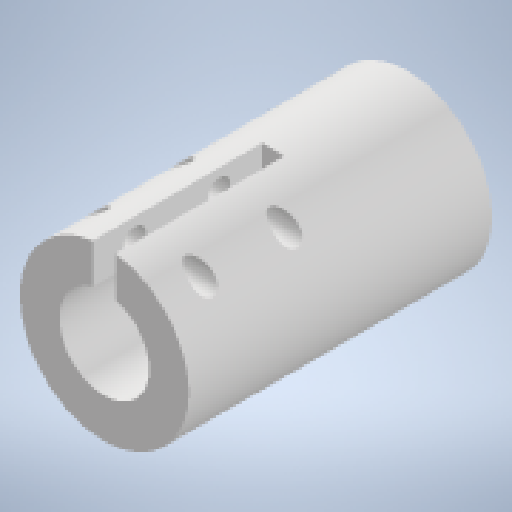
# Autodesk Inventor part: združevalnik_osi
Saved by Autodesk Inventor 2023 (Build 270158000, 158)
## iProperties
Created: 2022-09-16
Part Number: združevalnik_osi
Material: Generic
Document SubType Name: Modeling
Designer: simon
Density: 1 g/cm^3
Appearance: Default
Author: simon
Autodesk Inventor part; units mm, degrees
ref_plane "YZ Plane" through (0, 0, 0) normal (1, 0, 0) x (0, 1, 0)
ref_plane "XZ Plane" through (0, 0, 0) normal (0, 1, 0) x (-1, 0, 0)
ref_plane "XY Plane" through (0, 0, 0) normal (0, 0, 1) x (1, 0, 0)
sketch "Sketch1" plane through (0, 0, 0) normal (0, 0, 1) x (1, 0, 0)
  line L0 (-2.9047, -2.75) -> (-2.9047, 2.75) projected
  line L1 (-2.9047, 2.75) -> (2.9047, 2.75) projected
  line L2 (2.9047, 2.75) -> (2.9047, -2.75) projected
  line L3 (2.9047, -2.75) -> (-2.9047, -2.75) projected
  arc A0 (-7.5629, 23.8286) -> (-7.5205, 19.0707) centre (10.0684, 21.6064) ccw projected
  arc A1 (-7.5205, 19.0707) -> (-8.8044, 18.513) centre (0, 0) ccw projected
  arc A2 (-8.8044, 18.513) -> (-12.2528, 21.7915) centre (-22.663, 7.3892) ccw projected
  arc A3 (-12.2528, 21.7915) -> (-13.7113, 20.9046) centre (0, 0) ccw projected
  arc A4 (-13.7113, 20.9046) -> (-12.3868, 16.3345) centre (3.8657, 23.5216) ccw projected
  arc A5 (-12.3868, 16.3345) -> (-13.4727, 15.4511) centre (0, 0) ccw projected
  arc A6 (-13.4727, 15.4511) -> (-17.6777, 17.6777) centre (-23.8161, 1.0008) ccw projected
  arc A7 (-17.6777, 17.6777) -> (-18.8428, 16.4301) centre (0, 0) ccw projected
  arc A8 (-18.8428, 16.4301) -> (-16.3345, 12.3868) centre (-2.6237, 23.6923) ccw projected
  arc A9 (-16.3345, 12.3868) -> (-17.1417, 11.2433) centre (0, 0) ccw projected
  arc A10 (-17.1417, 11.2433) -> (-21.7915, 12.2528) centre (-23.203, -5.4619) ccw projected
  arc A11 (-21.7915, 12.2528) -> (-22.5769, 10.7371) centre (0, 0) ccw projected
  arc A12 (-22.5769, 10.7371) -> (-19.0707, 7.5205) centre (-8.9185, 22.1059) ccw projected
  arc A13 (-19.0707, 7.5205) -> (-19.5395, 6.2015) centre (0, 0) ccw projected
  arc A14 (-19.5395, 6.2015) -> (-24.2892, 5.9191) centre (-20.869, -11.5194) ccw projected
  arc A15 (-24.2892, 5.9191) -> (-24.6365, 4.2478) centre (0, 0) ccw projected
  arc A16 (-24.6365, 4.2478) -> (-20.3925, 2.0964) centre (-14.5519, 18.88) ccw projected
  arc A17 (-20.3925, 2.0964) -> (-20.488, 0.6999) centre (0, 0) ccw projected
  arc A18 (-20.488, 0.6999) -> (-24.9854, -0.8535) centre (-16.9872, -16.7226) ccw projected
  arc A19 (-24.9854, -0.8535) -> (-24.8689, -2.5566) centre (0, 0) ccw projected
  arc A20 (-24.8689, -2.5566) -> (-20.2019, -3.4832) centre (-19.106, 14.2538) ccw projected
  arc A21 (-20.2019, -3.4832) -> (-19.9171, -4.8537) centre (0, 0) ccw projected
  arc A22 (-19.9171, -4.8537) -> (-23.8286, -7.5629) centre (-11.8455, -20.6856) ccw projected
  arc A23 (-23.8286, -7.5629) -> (-23.257, -9.1714) centre (0, 0) ccw projected
  arc A24 (-23.257, -9.1714) -> (-18.513, -8.8044) centre (-22.2431, 8.5705) ccw projected
  arc A25 (-18.513, -8.8044) -> (-17.869, -10.0473) centre (0, 0) ccw projected
  arc A26 (-17.869, -10.0473) -> (-20.9046, -13.7113) centre (-5.8254, -23.1144) ccw projected
  arc A27 (-20.9046, -13.7113) -> (-19.9201, -15.1059) centre (0, 0) ccw projected
  arc A28 (-19.9201, -15.1059) -> (-15.4511, -13.4727) centre (-23.7306, 2.2515) ccw projected
  arc A29 (-15.4511, -13.4727) -> (-14.4957, -14.4957) centre (0, 0) ccw projected
  arc A30 (-14.4957, -14.4957) -> (-16.4301, -18.8428) centre (0.6268, -23.8289) ccw projected
  arc A31 (-16.4301, -18.8428) -> (-15.1059, -19.9201) centre (0, 0) ccw projected
  arc A32 (-15.1059, -19.9201) -> (-11.2433, -17.1417) centre (-23.4581, -4.2344) ccw projected
  arc A33 (-11.2433, -17.1417) -> (-10.0473, -17.869) centre (0, 0) ccw projected
  arc A34 (-10.0473, -17.869) -> (-10.7371, -22.5769) centre (7.0326, -22.7762) ccw projected
  arc A35 (-10.7371, -22.5769) -> (-9.1714, -23.257) centre (0, 0) ccw projected
  arc A36 (-9.1714, -23.257) -> (-6.2015, -19.5395) centre (-21.4457, -10.4063) ccw projected
  arc A37 (-6.2015, -19.5395) -> (-4.8537, -19.9171) centre (0, 0) ccw projected
  arc A38 (-4.8537, -19.9171) -> (-4.2478, -24.6365) centre (12.9167, -20.0342) ccw projected
  arc A39 (-4.2478, -24.6365) -> (-2.5566, -24.8689) centre (0, 0) ccw projected
  arc A40 (-2.5566, -24.8689) -> (-0.6999, -20.488) centre (-17.8429, -15.8064) ccw projected
  arc A41 (-0.6999, -20.488) -> (0.6999, -20.488) centre (0, 0) ccw projected
  arc A42 (0.6999, -20.488) -> (2.5566, -24.8689) centre (17.8429, -15.8064) ccw projected
  arc A43 (2.5566, -24.8689) -> (4.2478, -24.6365) centre (0, 0) ccw projected
  arc A44 (4.2478, -24.6365) -> (4.8537, -19.9171) centre (-12.9167, -20.0342) ccw projected
  arc A45 (4.8537, -19.9171) -> (6.2015, -19.5395) centre (0, 0) ccw projected
  arc A46 (6.2015, -19.5395) -> (9.1714, -23.257) centre (21.4457, -10.4063) ccw projected
  arc A47 (9.1714, -23.257) -> (10.7371, -22.5769) centre (0, 0) ccw projected
  arc A48 (10.7371, -22.5769) -> (10.0473, -17.869) centre (-7.0326, -22.7762) ccw projected
  arc A49 (10.0473, -17.869) -> (11.2433, -17.1417) centre (0, 0) ccw projected
  arc A50 (11.2433, -17.1417) -> (15.1059, -19.9201) centre (23.4581, -4.2344) ccw projected
  arc A51 (15.1059, -19.9201) -> (16.4301, -18.8428) centre (0, 0) ccw projected
  arc A52 (16.4301, -18.8428) -> (14.4957, -14.4957) centre (-0.6268, -23.8289) ccw projected
  arc A53 (14.4957, -14.4957) -> (15.4511, -13.4727) centre (0, 0) ccw projected
  arc A54 (15.4511, -13.4727) -> (19.9201, -15.1059) centre (23.7306, 2.2515) ccw projected
  arc A55 (19.9201, -15.1059) -> (20.9046, -13.7113) centre (0, 0) ccw projected
  arc A56 (20.9046, -13.7113) -> (17.869, -10.0473) centre (5.8254, -23.1144) ccw projected
  arc A57 (17.869, -10.0473) -> (18.513, -8.8044) centre (0, 0) ccw projected
  arc A58 (18.513, -8.8044) -> (23.257, -9.1714) centre (22.2431, 8.5705) ccw projected
  arc A59 (23.257, -9.1714) -> (23.8286, -7.5629) centre (0, 0) ccw projected
  arc A60 (23.8286, -7.5629) -> (19.9171, -4.8537) centre (11.8455, -20.6856) ccw projected
  arc A61 (19.9171, -4.8537) -> (20.2019, -3.4832) centre (0, 0) ccw projected
  arc A62 (20.2019, -3.4832) -> (24.8689, -2.5566) centre (19.106, 14.2538) ccw projected
  arc A63 (24.8689, -2.5566) -> (24.9854, -0.8535) centre (0, 0) ccw projected
  arc A64 (24.9854, -0.8535) -> (20.488, 0.6999) centre (16.9872, -16.7226) ccw projected
  arc A65 (20.488, 0.6999) -> (20.3925, 2.0964) centre (0, 0) ccw projected
  arc A66 (20.3925, 2.0964) -> (24.6365, 4.2478) centre (14.5519, 18.88) ccw projected
  arc A67 (24.6365, 4.2478) -> (24.2892, 5.9191) centre (0, 0) ccw projected
  arc A68 (24.2892, 5.9191) -> (19.5395, 6.2015) centre (20.869, -11.5194) ccw projected
  arc A69 (19.5395, 6.2015) -> (19.0707, 7.5205) centre (0, 0) ccw projected
  arc A70 (19.0707, 7.5205) -> (22.5769, 10.7371) centre (8.9185, 22.1059) ccw projected
  arc A71 (22.5769, 10.7371) -> (21.7915, 12.2528) centre (0, 0) ccw projected
  arc A72 (21.7915, 12.2528) -> (17.1417, 11.2433) centre (23.203, -5.4619) ccw projected
  arc A73 (17.1417, 11.2433) -> (16.3345, 12.3868) centre (0, 0) ccw projected
  arc A74 (16.3345, 12.3868) -> (18.8428, 16.4301) centre (2.6237, 23.6923) ccw projected
  arc A75 (18.8428, 16.4301) -> (17.6777, 17.6777) centre (0, 0) ccw projected
  arc A76 (17.6777, 17.6777) -> (13.4727, 15.4511) centre (23.8161, 1.0008) ccw projected
  arc A77 (13.4727, 15.4511) -> (12.3868, 16.3345) centre (0, 0) ccw projected
  arc A78 (12.3868, 16.3345) -> (13.7113, 20.9046) centre (-3.8657, 23.5216) ccw projected
  arc A79 (13.7113, 20.9046) -> (12.2528, 21.7915) centre (0, 0) ccw projected
  arc A80 (12.2528, 21.7915) -> (8.8044, 18.513) centre (22.663, 7.3892) ccw projected
  arc A81 (8.8044, 18.513) -> (7.5205, 19.0707) centre (0, 0) ccw projected
  arc A82 (7.5205, 19.0707) -> (7.5629, 23.8286) centre (-10.0684, 21.6064) ccw projected
  arc A83 (7.5629, 23.8286) -> (5.9191, 24.2892) centre (0, 0) ccw projected
  arc A84 (5.9191, 24.2892) -> (3.4832, 20.2019) centre (19.829, 13.2296) ccw projected
  arc A85 (3.4832, 20.2019) -> (2.0964, 20.3925) centre (0, 0) ccw projected
  arc A86 (2.0964, 20.3925) -> (0.8535, 24.9854) centre (-15.5244, 18.0888) ccw projected
  arc A87 (0.8535, 24.9854) -> (-0.8535, 24.9854) centre (0, 0) ccw projected
  arc A88 (-0.8535, 24.9854) -> (-2.0964, 20.3925) centre (15.5244, 18.0888) ccw projected
  arc A89 (-2.0964, 20.3925) -> (-3.4832, 20.2019) centre (0, 0) ccw projected
  arc A90 (-3.4832, 20.2019) -> (-5.9191, 24.2892) centre (-19.829, 13.2296) ccw projected
  arc A91 (-5.9191, 24.2892) -> (-7.5629, 23.8286) centre (0, 0) ccw projected
  circle A92 centre (0, 0) radius 7.5
  point P0 (0, 0)
  dimension "d0" = 15
  constraints: 1 centre point, 1 coincident
  measures "d0" diameter of A92
extrude "Extrusion1" add sketch "Sketch1" along normal blind 12 contours A92
sketch "Sketch2" plane through (0, 0, 12) normal (0, 0, 1) x (1, 0, 0)
  circle A0 centre (0, 0) radius 7.5 projected
  line L0 (-2.9047, -2.75) -> (-2.9047, 2.75) projected
  line L1 (-2.9047, 2.75) -> (2.9047, 2.75) projected
  line L2 (2.9047, 2.75) -> (2.9047, -2.75) projected
  line L3 (2.9047, -2.75) -> (-2.9047, -2.75) projected
  circle A1 centre (0, 0) radius 4
  line L4 (1, 7.5) -> (-1, 7.5)
  line L5 (-1, 7.5) -> (-1, -7.5)
  line L6 (-1, -7.5) -> (1, -7.5)
  line L7 (1, -7.5) -> (1, 7.5)
  line L8 (1, 7.5) -> (-1, -7.5) construction
  line L9 (-1, 7.5) -> (1, -7.5) construction
  point P0 (0, 0)
  point P1 (-1, -7.433)
  point P2 (-1, -3.873)
  point P3 (-1, 3.873)
  point P4 (-1, 7.433)
  point P5 (1, 7.433)
  point P6 (1, 3.873)
  point P7 (1, -3.873)
  point P8 (1, -7.433)
  dimension "d3" = 8
  dimension "d4" = 2
  dimension "d5" = 15
  constraints: 12 end point, 2 midpoint, 2 parallel, 1 centre point, 1 coincident, 1 horizontal, 1 perpendicular
  measures "d3" diameter of A1
  measures "d4" distance of L6.end L5.end
  measures "d5" distance of L5.end L4.end
extrude "Extrusion2" add sketch "Sketch2" along normal blind 15 contours A0 L7 A1 | A0 L5 A1 L7 | L5 A1 A0 picked at (0, -5.1572)
sketch "Sketch3" plane through (-1, 3.873, 12) normal (1, 0, 0) x (0, 0, -1)
  line L0 (0, 3.5601) -> (0, 3.5601) projected
  line L1 (12, 3.627) -> (12, -11.373) projected
  line L2 (0, -1.123) -> (0, 0) projected
  line L3 (0, -6.623) -> (0, -1.123) projected
  line L4 (0, -6.623) -> (0, -6.623) projected
  line L5 (0, -1.123) -> (0, -6.623) projected
  line L6 (0, 0) -> (0, -1.123) projected
  line L7 (0, 0) -> (-15, 0) projected
  line L8 (-15, 0) -> (-15, 0) projected
  line L9 (0, 0) -> (-15, 0) projected
  line L10 (0, 0) -> (-15, 0)
  line L11 (-15, 0) -> (-15, 2.0431)
  line L12 (0, 2.0431) -> (0, 0)
  line L13 (0, 3.5601) -> (-15, 3.5601) projected
  line L14 (-15, 3.5601) -> (-15, 3.5601) projected
  line L15 (0, 3.5601) -> (-15, 3.5601) projected
  line L16 (0, 0) -> (-15, 3.5601)
  line L17 (-7.5, 1.78) -> (-15, 1.78)
  line L18 (-7.5, 1.78) -> (0, 1.78)
  circle A0 centre (-3.75, 1.78) radius 1
  circle A1 centre (-11.25, 1.78) radius 1
  point P0 (12, -3.873)
  point P1 (0, -11.373)
  point P2 (0, 3.627)
  dimension "d8" = 2
  dimension "d9" = 2
  constraints: 12 end point, 3 midpoint, 3 point on line, 2 centre point, 2 perpendicular, 1 horizontal, 1 parallel
  measures "d8" diameter of A0
  measures "d9" diameter of A1
extrude "Extrusion3" cut sketch "Sketch3" along normal mid plane 15 contours A0 L16 | L16 A0 L18 | L18 A0 | A1 L16 L17 | L17 A1 | A1 L16 picked at (-4.0561, 1.6481) picked at (-11.0212, 2.0224)
body "Solid1"
